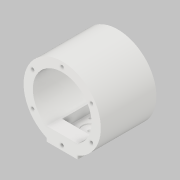
# Autodesk Inventor part: SJ003
Saved by Autodesk Inventor 2017 (Build 210142000, 142)
## iProperties
Created: 2017-06-01
Part Number: SJ003
Material: ABS Plastic
Document SubType Name: Modeling
Designer: Zach
Density: 1.06 g/cm^3
Appearance: CR White
Author: Zach
Autodesk Inventor part; units mm, degrees
ref_plane "YZ Plane" through (0, 0, 0) normal (1, 0, 0) x (0, 1, 0)
ref_plane "XZ Plane" through (0, 0, 0) normal (0, 1, 0) x (-1, 0, 0)
ref_plane "XY Plane" through (0, 0, 0) normal (0, 0, 1) x (1, 0, 0)
sketch "Sketch1" plane through (0, 0, 0) normal (0, 0, 1) x (1, 0, 0)
  circle A0 centre (0, 0) radius 62.5
  circle A1 centre (0, 0) radius 47.5
  dimension "d0" = 125
  dimension "d1" = 15
  constraints: 2 centre point, 1 coincident
  measures "d0" diameter of A0
  measures "d1" radial gap between concentric circles of A0 A1
extrude "Extrusion1" add sketch "Sketch1" along normal mid plane 90
sketch "Sketch3" plane through (0, 0, 45) normal (0, 0, 1) x (1, 0, 0)
  line L0 (25, -40.3887) -> (25, -62.5)
  line L1 (25, -62.5) -> (-25, -62.5)
  line L2 (-25, -62.5) -> (-25, -40.3887)
  line L3 (-25, -40.3887) -> (25, -40.3887)
  circle A0 centre (0, 0) radius 62.5 projected
  circle A1 centre (0, 0) radius 47.5 projected
  circle A2 centre (0, 0) radius 62.5 projected
  circle A3 centre (0, 0) radius 47.5 projected
  point P0 (0, -62.5)
  dimension "d17" = 25
  dimension "d18" = 50
  constraints: 8 end point, 2 perpendicular, 1 horizontal, 1 midpoint, 1 vertical, 1 vertical alignment, 3 other
  measures "d17" horizontal distance of L2.end point (0, 0)
  measures "d18" distance of L2.end L0.start
extrude "Extrusion3" add sketch "Sketch3" against normal blind 90 contours A1 L3 | L0 A0 L2 A1 | L0 L1 A0 | L1 L2 A0 picked at (-5.7183, -41.6905) picked at (14.2711, -50.3828)
sketch "Sketch2" plane through (0, 0, 45) normal (0, 0, 1) x (1, 0, 0)
  circle A0 centre (0, 55) radius 2.5
  circle A1 centre (-47.6314, 27.5) radius 2.5
  circle A2 centre (-47.6314, -27.5) radius 2.5
  circle A3 centre (0, -55) radius 2.5
  circle A4 centre (47.6314, -27.5) radius 2.5
  circle A5 centre (47.6314, 27.5) radius 2.5
  point P0 (0, 0)
  dimension "d4" = 5
  dimension "d5" = 55
  dimension "d8" = 360
  constraints: 6 centre point, 13 other
  measures "d4" diameter of A0
  measures "d5" distance of point (0, 0) A0.centre
extrude "Extrusion2" cut sketch "Sketch2" against normal through all
sketch "Sketch5" plane through (-25, -40.3887, 45) normal (0, 1, 0) x (1, 0, 0)
  line L0 (2.5, 67.5) -> (47.5, 67.5)
  line L1 (47.5, 67.5) -> (47.5, 22.5)
  line L2 (47.5, 22.5) -> (2.5, 22.5)
  line L3 (2.5, 22.5) -> (2.5, 67.5)
  line L4 (2.5, 67.5) -> (47.5, 22.5) construction
  line L5 (47.5, 67.5) -> (2.5, 22.5) construction
  line L6 (0, 0) -> (50, 0) projected
  line L7 (0, 0) -> (0, 90) projected
  line L8 (50, 90) -> (0, 90) projected
  line L9 (50, 0) -> (50, 90) projected
  point P0 (25, 45)
  dimension "d10" = 120
  dimension "d20" = 45
  dimension "d21" = 45
  dimension "d57" = 45
  dimension "d58" = 2.5
  constraints: 12 end point, 2 midpoint, 2 parallel, 1 horizontal, 1 perpendicular
  measures "d20" distance of L1.end L2.end
  measures "d21" distance of L0.end L1.end
  measures "d57" distance from line of L8 point (25, 45)
  measures "d58" distance between parallel lines of L3 L7
extrude "Extrusion4" cut sketch "Sketch5" against normal blind 15 contours L0 L1 L2 L3
sketch "Sketch6" plane through (-25, -55.3887, 45) normal (0, 1, 0) x (1, 0, 0)
  line L0 (40.5, 29.5) -> (9.5, 29.5) construction
  line L1 (9.5, 29.5) -> (9.5, 60.5) construction
  line L2 (9.5, 60.5) -> (40.5, 60.5) construction
  line L3 (40.5, 60.5) -> (40.5, 29.5) construction
  line L4 (40.5, 29.5) -> (9.5, 60.5) construction
  line L5 (9.5, 29.5) -> (40.5, 60.5) construction
  circle A0 centre (9.5, 60.5) radius 1.65
  circle A1 centre (40.5, 60.5) radius 1.65
  circle A2 centre (40.5, 29.5) radius 1.65
  circle A3 centre (9.5, 29.5) radius 1.65
  circle A4 centre (25, 45) radius 3
  dimension "d24" = 31
  dimension "d25" = 31
  dimension "d26" = 3.3
  dimension "d27" = 3.3
  dimension "d28" = 3.3
  dimension "d29" = 3.3
  dimension "d32" = 6
  constraints: 12 end point, 5 centre point, 5 coincident, 2 midpoint, 2 parallel, 1 horizontal, 1 perpendicular
  measures "d24" distance of L0.end L1.end
  measures "d25" distance of L1.end L2.end
  measures "d26" diameter of A0
  measures "d27" diameter of A1
  measures "d28" diameter of A2
  measures "d29" diameter of A3
  measures "d32" diameter of A4
extrude "Extrusion5" cut sketch "Sketch6" against normal through all
sketch "Sketch8" plane through (-25, -55.3887, 45) normal (0, 1, 0) x (1, 0, 0)
  circle A0 centre (25, 45) radius 12.5
  dimension "d38" = 25
  constraints: 1 centre point, 1 coincident
  measures "d38" diameter of A0
extrude "Extrusion7" cut sketch "Sketch8" against normal blind 2
body "Solid1"
